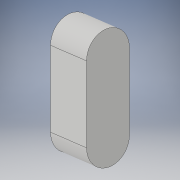
# Autodesk Inventor part: Component 17 (Feather Key)
Saved by Autodesk Inventor 2018 (Build 220112000, 112)
## iProperties
Created: 2023-03-15
Part Number: Component 17 (Feather Key)
Material: Generic
Document SubType Name: Modeling
Designer: Habib Mohamed
Density: 1 g/cm^3
Appearance: Default
Author: Habib Mohamed
Autodesk Inventor part; units mm, degrees
ref_plane "YZ Plane" through (0, 0, 0) normal (1, 0, 0) x (0, 1, 0)
ref_plane "XZ Plane" through (0, 0, 0) normal (0, 1, 0) x (-1, 0, 0)
ref_plane "XY Plane" through (0, 0, 0) normal (0, 0, 1) x (1, 0, 0)
sketch "Sketch1" plane through (0, 0, 0) normal (1, 0, 0) x (0, 1, 0)
  line L0 (2.5, 0) -> (-2.5, 0) construction
  line L1 (2.5, 1.5) -> (-2.5, 1.5)
  line L2 (-2.5, -1.5) -> (2.5, -1.5)
  arc A0 (2.5, -1.5) -> (2.5, 1.5) centre (2.5, 0) ccw
  arc A1 (-2.5, 1.5) -> (-2.5, -1.5) centre (-2.5, 0) ccw
  point P0 (0, 0)
  point P1 (0, 0)
  dimension "d0" = 1.5
  dimension "d1" = 5
  constraints: 8 end point, 4 point on circle, 4 tangent, 2 centre point, 1 coincident, 1 horizontal, 1 midpoint, 1 parallel
  measures "d0" radius of A0
  measures "d1" distance of L0.start L0.end
extrude "Extrusion1" add sketch "Sketch1" along normal blind 3
body "Solid1"
